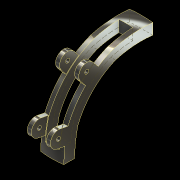
# Autodesk Inventor part: New_part4
Saved by Autodesk Inventor 2016 (Build 200138000, 138)
## iProperties
Created: 2020-11-30
Part Number: New_part4
Material: 은
Document SubType Name: Modeling
Designer: Administrator
Density: 10.49 g/cm^3
Appearance: 은
Author: Administrator
Autodesk Inventor part; units mm, degrees
ref_plane "YZ Plane" through (0, 0, 0) normal (1, 0, 0) x (0, 1, 0)
ref_plane "XZ Plane" through (0, 0, 0) normal (0, 1, 0) x (-1, 0, 0)
ref_plane "XY Plane" through (0, 0, 0) normal (0, 0, 1) x (1, 0, 0)
sketch "스케치2" plane through (0, 0, 0) normal (0, 0, 1) x (1, 0, 0)
  line L0 (0, -100) -> (0, 100)
  circle A0 centre (0, 0) radius 100
  dimension "d2" = 200
  constraints: 2 end point, 2 point on circle, 1 centre point, 1 vertical
  measures "d2" diameter of A0
sketch "스케치2 outline for 회전1" plane through (0, 0, 0) normal (0, 0, 1) x (1, 0, 0)
  arc A0 (0, -100) -> (0, 100) centre (0, 0) ccw
  line L0 (0, 100) -> (0, -100)
revolve "회전1" add sketch "스케치2 outline for 회전1" angle 180 about axis through (0, -100, 0) along (0, -1, 0)
sketch "스케치4" plane through (0, 0, 0) normal (0, 1, 0) x (-1, 0, 0)
  line L0 (0, 0) -> (100, 0)
  line L1 (0, 5.96) -> (99.822234, 5.96)
  arc A0 (100, 0) -> (99.822234, 5.96) centre (0, 0) ccw
  line L2 (0, 0) -> (0, -101.396229)
  line L3 (0, 0) -> (0, 5.96)
  constraints: 8 end point, 2 point on circle, 1 centre point, 1 horizontal, 1 parallel, 1 vertical
sketch "스케치4 outline for 회전2" plane through (0, 0, 0) normal (0, 1, 0) x (-1, 0, 0)
  line L0 (100, 0) -> (0, 0)
  line L1 (0, 0) -> (0, 5.96)
  line L2 (0, 5.96) -> (99.822234, 5.96)
  arc A0 (99.822234, 5.96) -> (100, 0) centre (0, 0) cw
revolve "회전2" cut sketch "스케치4 outline for 회전2" angle 360 about axis through (0, 0, 0) along (0, 0, -1)
sketch "스케치5" plane through (0, 0, 0) normal (0, 1, 0) x (-1, 0, 0)
  arc A0 (99.822234, 5.96) -> (0, 100) centre (0, 0) ccw
  arc A1 (64.260394, 47.114532) -> (25.509602, 86.309097) centre (-0.44, 21.9) ccw
  arc A2 (66.824386, 5.96) -> (64.260394, 47.114532) centre (-56.08, 18.96) ccw
  arc A3 (25.509602, 86.309097) -> (0, 90) centre (0, 0) ccw
  line L0 (0, 5.96) -> (0, -74.633703)
  line L1 (66.336158, 0) -> (66.04701, 0)
  line L2 (66.824386, 5.96) -> (99.822234, 5.96)
  line L3 (0, 90) -> (0, 100)
  point P0 (-66.336158, 0)
  point P1 (-68.025723, 5.96)
  constraints: 10 point on circle, 8 end point, 4 centre point, 2 vertical, 1 horizontal, 1 point on line
sketch "스케치5 outline for 회전4" plane through (0, 0, 0) normal (0, 1, 0) x (-1, 0, 0)
  line L0 (66.824386, 5.96) -> (99.822234, 5.96)
  arc A0 (64.260394, 47.114532) -> (66.824386, 5.96) centre (-56.08, 18.96) cw
  arc A1 (25.509602, 86.309097) -> (64.260394, 47.114532) centre (-0.44, 21.9) cw
  arc A2 (0, 90) -> (25.509602, 86.309097) centre (0, 0) cw
  line L1 (0, 100) -> (0, 90)
  arc A3 (99.822234, 5.96) -> (0, 100) centre (0, 0) ccw
revolve "회전4" cut sketch "스케치5 outline for 회전4" angle 360 about axis through (0, 0, 5.96) along (0, 0, -1)
sketch "스케치6" plane through (0, 0, 0) normal (1, 0, 0) x (0, 1, 0)
  arc A0 (-67.493816, 20.96) -> (-66.824386, 5.96) centre (56.08, 18.96) ccw
  line L0 (66.824386, 5.96) -> (-66.824386, 5.96)
  arc A1 (25.509602, 86.309097) -> (10, 89.442719) centre (0, 0) ccw
  arc A2 (66.824386, 5.96) -> (64.260394, 47.114532) centre (-56.08, 18.96) ccw
  arc A3 (64.260394, 47.114532) -> (25.509602, 86.309097) centre (-0.44, 21.9) ccw
  arc A4 (-54.685783, 44.131995) -> (-57.492391, 20.96) centre (56.08, 18.96) ccw
  arc A5 (-22.211572, 76.854707) -> (-54.685783, 44.131995) centre (0.44, 21.9) ccw
  arc A6 (10, 79.372539) -> (-22.211572, 76.854707) centre (0, 0) ccw
  line L1 (10, 79.372539) -> (10, 89.442719)
  arc A7 (-63.799925, 48.265615) -> (-64.260394, 47.114532) centre (0.44, 21.9) ccw
  line L2 (-67.493816, 20.96) -> (-57.492391, 20.96)
  constraints: 17 point on circle, 8 centre point, 6 end point
sketch "스케치6 outline for 돌출1" plane through (0, 0, 0) normal (1, 0, 0) x (0, 1, 0)
  arc A0 (10, 89.442719) -> (25.509602, 86.309097) centre (0, 0) cw
  arc A1 (25.509602, 86.309097) -> (64.260394, 47.114532) centre (-0.44, 21.9) cw
  arc A2 (64.260394, 47.114532) -> (66.824386, 5.96) centre (-56.08, 18.96) cw
  line L0 (66.824386, 5.96) -> (-66.824386, 5.96)
  arc A3 (-66.824386, 5.96) -> (-67.493816, 20.96) centre (56.08, 18.96) cw
  line L1 (-67.493816, 20.96) -> (-57.492391, 20.96)
  arc A4 (-57.492391, 20.96) -> (-54.685783, 44.131995) centre (56.08, 18.96) cw
  arc A5 (-54.685783, 44.131995) -> (-22.211572, 76.854707) centre (0.44, 21.9) cw
  arc A6 (-22.211572, 76.854707) -> (10, 79.372539) centre (0, 0) cw
  line L2 (10, 79.372539) -> (10, 89.442719)
extrude "돌출1" cut sketch "스케치6 outline for 돌출1" along normal mid plane 140
sketch "스케치7" plane through (0, 0, 0) normal (0, 1, 0) x (-1, 0, 0)
  line L0 (-10, 20.96) -> (-10, 89.442719)
  arc A0 (-25.509602, 86.309097) -> (-68.993637, 20.96) centre (0.44, 21.9) ccw
  line L1 (-10, 20.96) -> (-68.993637, 20.96)
  arc A1 (-10, 89.442719) -> (-25.509602, 86.309097) centre (0, 0) ccw
  line L2 (10, 20.96) -> (10, 89.442719)
  arc A2 (68.993637, 20.96) -> (25.509602, 86.309097) centre (-0.44, 21.9) ccw
  line L3 (10, 20.96) -> (68.993637, 20.96)
  arc A3 (25.509602, 86.309097) -> (10, 89.442719) centre (0, 0) ccw
  point P0 (-35.355907, 20.96)
  point P1 (35.355907, 20.96)
  constraints: 8 end point, 8 point on circle, 4 centre point, 1 coincident, 1 horizontal
sketch "스케치7 outline for 돌출2" plane through (0, 0, 0) normal (0, 1, 0) x (-1, 0, 0)
  line L0 (-68.993637, 20.96) -> (-10, 20.96)
  arc A0 (-25.509602, 86.309097) -> (-68.993637, 20.96) centre (0.44, 21.9) ccw
  arc A1 (-10, 89.442719) -> (-25.509602, 86.309097) centre (0, 0) ccw
  line L1 (-10, 20.96) -> (-10, 89.442719)
  line L2 (10, 20.96) -> (10, 89.442719)
  arc A2 (10, 89.442719) -> (25.509602, 86.309097) centre (0, 0) cw
  arc A3 (25.509602, 86.309097) -> (68.993637, 20.96) centre (-0.44, 21.9) cw
  line L3 (68.993637, 20.96) -> (10, 20.96)
extrude "돌출2" cut sketch "스케치7 outline for 돌출2" along normal mid plane 140
sketch "스케치8" plane through (10, -66.748897, 20.96) normal (1, 0, 0) x (0, 0, -1)
  line L0 (-57.722456, 30.299383) -> (-48.923751, 19.40981)
  line L1 (-63.945069, 25.271551) -> (-57.722456, 30.299383)
  circle A0 centre (-59.545716, 19.826765) radius 1.75
  line L2 (-55.146364, 14.381979) -> (-48.923751, 19.40981)
  arc A1 (-63.945069, 25.271551) -> (-55.146364, 14.381979) centre (-59.545716, 19.826765) ccw
  line L3 (-49.701578, 18.781331) -> (-58.500282, 29.670904)
  circle A2 centre (-21.454312, -4.589059) radius 1.75
  arc A3 (-28.327325, -3.26177) -> (-14.5813, -5.916347) centre (-21.454312, -4.589059) ccw
  line L4 (-28.327325, -3.26177) -> (-26.810424, 4.593102)
  line L5 (-14.5813, -5.916347) -> (-13.064398, 1.938524)
  line L6 (-26.810424, 4.593102) -> (-13.064398, 1.938524)
  line L7 (-13.254011, 0.956665) -> (-27.000036, 3.611243)
  constraints: 16 end point, 4 centre point, 4 point on circle, 4 point on line, 2 coincident
sketch "스케치8 outline for 돌출3" plane through (10, -66.748897, 20.96) normal (1, 0, 0) x (0, 0, -1)
  line L0 (-58.500282, 29.670904) -> (-63.945069, 25.271551)
  line L1 (-49.701578, 18.781331) -> (-58.500282, 29.670904)
  arc A0 (-63.945069, 25.271551) -> (-55.146364, 14.381979) centre (-59.545716, 19.826765) ccw
  line L2 (-55.146364, 14.381979) -> (-49.701578, 18.781331)
  circle A1 centre (-59.545716, 19.826765) radius 1.75
  arc A2 (-28.327325, -3.26177) -> (-14.5813, -5.916347) centre (-21.454312, -4.589059) ccw
  line L3 (-27.000036, 3.611243) -> (-28.327325, -3.26177)
  line L4 (-14.5813, -5.916347) -> (-13.254011, 0.956665)
  line L5 (-13.254011, 0.956665) -> (-27.000036, 3.611243)
  circle A3 centre (-21.454312, -4.589059) radius 1.75
extrude "돌출3" add sketch "스케치8 outline for 돌출3" against normal blind 3.5
sketch "스케치9" plane through (-10, -66.748897, 20.96) normal (-1, 0, 0) x (0, 0, 1)
  line L0 (57.722456, 30.299383) -> (48.923751, 19.40981)
  line L1 (63.945069, 25.271551) -> (57.722456, 30.299383)
  circle A0 centre (59.545716, 19.826765) radius 1.75
  line L2 (55.146364, 14.381979) -> (48.923751, 19.40981)
  arc A1 (55.146364, 14.381979) -> (63.945069, 25.271551) centre (59.545716, 19.826765) ccw
  line L3 (49.701578, 18.781331) -> (58.500282, 29.670904)
  circle A2 centre (21.454312, -4.589059) radius 1.75
  arc A3 (14.5813, -5.916347) -> (28.327325, -3.26177) centre (21.454312, -4.589059) ccw
  line L4 (28.327325, -3.26177) -> (26.810424, 4.593102)
  line L5 (14.5813, -5.916347) -> (13.064398, 1.938524)
  line L6 (26.810424, 4.593102) -> (13.064398, 1.938524)
  line L7 (13.254011, 0.956665) -> (27.000036, 3.611243)
  constraints: 16 end point, 4 centre point, 4 point on circle, 4 point on line, 2 coincident
sketch "스케치9 outline for 돌출4" plane through (-10, -66.748897, 20.96) normal (-1, 0, 0) x (0, 0, 1)
  arc A0 (55.146364, 14.381979) -> (63.945069, 25.271551) centre (59.545716, 19.826765) ccw
  line L0 (49.701578, 18.781331) -> (55.146364, 14.381979)
  line L1 (63.945069, 25.271551) -> (58.500282, 29.670904)
  line L2 (58.500282, 29.670904) -> (49.701578, 18.781331)
  circle A1 centre (59.545716, 19.826765) radius 1.75
  line L3 (13.254011, 0.956665) -> (14.5813, -5.916347)
  line L4 (27.000036, 3.611243) -> (13.254011, 0.956665)
  arc A2 (14.5813, -5.916347) -> (28.327325, -3.26177) centre (21.454312, -4.589059) ccw
  line L5 (28.327325, -3.26177) -> (27.000036, 3.611243)
  circle A3 centre (21.454312, -4.589059) radius 1.75
extrude "돌출4" add sketch "스케치9 outline for 돌출4" against normal blind 3.5
sketch "스케치11" plane through (0, 0, 0) normal (1, 0, 0) x (0, 1, 0)
  line L0 (-3.150132, 29.959716) -> (-3.150132, 99.501587)
  line L1 (-19.150132, 99.501587) -> (-3.150132, 99.501587)
  line L2 (-3.150132, 29.959716) -> (-82.78397, 29.959716)
  line L3 (-82.78397, 45.959716) -> (-82.78397, 29.959716)
  line L4 (-82.78397, 45.959716) -> (-19.150132, 99.501587)
  point P0 (-11.150132, 37.959716)
  constraints: 10 end point, 1 horizontal, 1 vertical
sketch "스케치11 outline for 돌출5" plane through (0, 0, 0) normal (1, 0, 0) x (0, 1, 0)
  line L0 (-3.150132, 99.501587) -> (-3.150132, 29.959716)
  line L1 (-3.150132, 29.959716) -> (-82.78397, 29.959716)
  line L2 (-82.78397, 29.959716) -> (-82.78397, 45.959716)
  line L3 (-82.78397, 45.959716) -> (-19.150132, 99.501587)
  line L4 (-19.150132, 99.501587) -> (-3.150132, 99.501587)
extrude "돌출5" cut sketch "스케치11 outline for 돌출5" along normal mid plane 12
